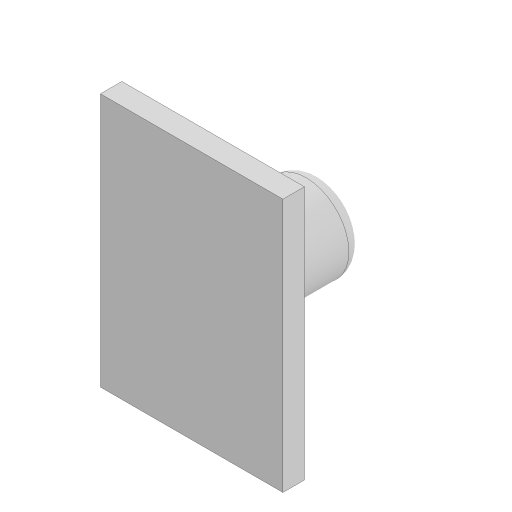
# Autodesk Inventor part: tombol
Saved by Autodesk Inventor 2023 (Build 270158000, 158)
## iProperties
Created: 2025-11-27
Part Number: tombol
Material: Generic
Document SubType Name: Modeling
Designer: dinoo
Density: 1 g/cm^3
Appearance: Default
Author: dinoo
Autodesk Inventor part; units mm, degrees
ref_plane "YZ Plane" through (0, 0, 0) normal (1, 0, 0) x (0, 1, 0)
ref_plane "XZ Plane" through (0, 0, 0) normal (0, 1, 0) x (-1, 0, 0)
ref_plane "XY Plane" through (0, 0, 0) normal (0, 0, 1) x (1, 0, 0)
sketch "Sketch1" plane through (0, 0, 0) normal (0, 0, 1) x (1, 0, 0)
  line L0 (2.554, -3.555) -> (-2.554, -3.555)
  line L1 (-2.554, -3.555) -> (-2.554, 3.555)
  line L2 (-2.554, 3.555) -> (2.554, 3.555)
  line L3 (2.554, 3.555) -> (2.554, -3.555)
  line L4 (2.554, -3.555) -> (-2.554, 3.555) construction
  line L5 (-2.554, -3.555) -> (2.554, 3.555) construction
  point P0 (0, 0)
  dimension "d0" = 5.108
  dimension "d1" = 7.11
  constraints: 12 end point, 2 midpoint, 2 parallel, 1 horizontal, 1 perpendicular
  measures "d0" distance of L1.end L2.end
  measures "d1" distance of L0.end L1.end
sketch "Sketch2" plane through (0, 0, 0) normal (0, 0, 1) x (1, 0, 0)
  circle A0 centre (0, 0) radius 1.2
  dimension "d2" = 2.4
  constraints: 1 centre point, 1 coincident
  measures "d2" diameter of A0
extrude "Extrusion1" add sketch "Sketch1" along normal blind 0.6
extrude "Extrusion2" add sketch "Sketch2" against normal blind 3
fillet "Fillet1" radius 0.4 1 edges at (-1.2, 0, -3)
body "Solid1"
